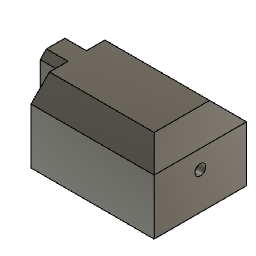
Finger tip v1 (Autodesk Fusion 360 design; units mm, degrees)
Autodesk Fusion 360 part; units mm, degrees
sketch "Sketch1" plane through (0, 0, 0) normal (0, 0, 1) x (1, 0, 0)
  line L0 (0, 0) -> (20, 0)
  line L1 (20, 0) -> (20, 15)
  line L2 (20, 15) -> (0, 15)
  line L3 (0, 15) -> (0, 0)
  dimension "d1" = 15
  constraint coincident L0.start L3.end
  constraint horizontal L0
  constraint perpendicular L0 L1
  constraint perpendicular L1 L2
  constraint perpendicular L0 L3
  measures "d1" distance of L0.end L1.end
sketch "Sketch2" plane through (0, 0, 0) normal (0, 0, 1) x (1, 0, 0)
  line L0 (0, 10) -> (-3.5, 10)
  line L1 (-3.5, 10) -> (-3.5, 5)
  line L2 (-3.5, 5) -> (0, 5)
  line L3 (0, 5) -> (0, 10)
  dimension "d2" = 3.5
  constraint horizontal L0
  constraint perpendicular L0 L1
  constraint perpendicular L1 L2
  constraint perpendicular L0 L3
  measures "d2" distance of L0.start L0.end
extrude "Extrude1" add sketch "Sketch1" sketch "Sketch2" along normal blind 12 of sketch 2
chamfer "Chamfer1" distance 3 angle 45 1 edges at (10, 0, 12)
chamfer "Chamfer2" distance 3 angle 45 1 edges at (10, 15, 12)
hole "Hole1" at (-1.75, 5, 6) direction (0, 1, 0) diameter 2.5 depth 9 tip angle 118
hole "Hole2" at (20, 7.5, 6) direction (-1, 0, 0) diameter 1.75 depth 38 tip angle 118
chamfer "Chamfer3" distance 3 angle 45 1 edges at (20, 7.5, 12)
chamfer "Chamfer4" distance 1 angle 45 2 edges at (-1.75, 5, 12) (-1.75, 10, 12)
